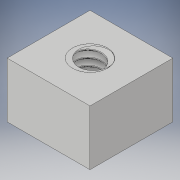
# Autodesk Inventor part: Nut0.25-20
Saved by Autodesk Inventor 2019 (Build 230136000, 136)
## iProperties
Created: 2019-08-02
Part Number: Nut0.25-20
Material: Generic
Document SubType Name: Modeling
Designer: aorfi
Density: 1 g/cm^3
Appearance: Default
Author: aorfi
Autodesk Inventor part; units mm, degrees
ref_plane "YZ Plane" through (0, 0, 0) normal (1, 0, 0) x (0, 1, 0)
ref_plane "XZ Plane" through (0, 0, 0) normal (0, 1, 0) x (-1, 0, 0)
ref_plane "XY Plane" through (0, 0, 0) normal (0, 0, 1) x (1, 0, 0)
sketch "Sketch1" plane through (0, 0, 0) normal (0, 1, 0) x (-1, 0, 0)
  line L0 (-7.5, 7.5) -> (7.5, 7.5)
  line L1 (7.5, 7.5) -> (7.5, -7.5)
  line L2 (7.5, -7.5) -> (-7.5, -7.5)
  line L3 (-7.5, -7.5) -> (-7.5, 7.5)
  line L4 (-7.5, 7.5) -> (7.5, -7.5) construction
  line L5 (7.5, 7.5) -> (-7.5, -7.5) construction
  point P0 (0, 0)
  dimension "d0" = 15
  dimension "d1" = 15
  constraints: 12 end point, 2 midpoint, 2 parallel, 1 horizontal, 1 perpendicular
  measures "d0" distance of L0.end L1.end
  measures "d1" distance of L1.end L2.end
extrude "Extrusion1" add sketch "Sketch1" along normal mid plane 10
sketch "Sketch2" plane through (0, 5, 0) normal (0, 1, 0) x (1, 0, 0)
  circle A0 centre (0, 0) radius 3.175
  dimension "d4" = 6.35
  constraints: 1 centre point, 1 coincident
  measures "d4" diameter of A0
extrude "Extrusion2" cut sketch "Sketch2" against normal blind 10
thread "Thread1" size "1/4-20 UNC" class "2B" standard "ANSI Unified Screw Threads" full length
sketch "Sketch4" plane through (0, -5, 0) normal (-1, 0, 0) x (0, 0, 1)
  line L0 (3.175, 0) -> (3.175, 10)
  line L1 (3.175, 10) -> (2.2333, 10)
  line L2 (2.2333, 10) -> (2.2333, 0)
  line L3 (2.2333, 0) -> (3.175, 0)
  line L4 (0, -3.6619) -> (0, 12.277) projected
  constraints: 8 end point
revolve "Revolution1" add sketch "Sketch4" angle 360 about axis through (0, -5, 0) along (0, 1, 0) separate body
sketch "Sketch3" plane through (0, -5, 3.175) normal (1, 0, 0) x (0, 1, 0)
  line L0 (-0.7409, -0.0644) -> (-0.6351, -0.0644) construction
  line L1 (0.1057, -0.8776) -> (-0.0001, -1.0809) construction
  line L2 (-1.2701, -1.0809) -> (-1.3759, -0.8776) construction
  line L3 (-0.5293, -0.0644) -> (-0.6351, 0.1389) construction
  line L4 (-0.6351, 0.1389) -> (-0.7409, -0.0644) construction
  line L5 (-1.2701, -1.0809) -> (-1.1643, -0.8776) construction
  line L6 (-0.5293, -0.0644) -> (-0.1059, -0.8776)
  line L7 (-1.3759, -0.8776) -> (-1.1643, -0.8776) construction
  arc A0 (-1.3759, -0.8776) -> (-1.2701, -0.9418) centre (-1.2701, -0.8225) ccw construction
  line L8 (0.1057, -0.8776) -> (-0.1059, -0.8776) construction
  line L9 (-1.2701, -1.0809) -> (-1.2701, -0.8776) construction
  line L10 (-0.0001, -1.0809) -> (-0.0001, -0.8776) construction
  line L11 (-0.6351, 0.1389) -> (-0.6351, -0.0002) construction
  line L12 (-1.2701, -0.9418) -> (-0.0001, -0.9418)
  arc A1 (-1.2701, -0.9418) -> (-1.1643, -0.8776) centre (-1.2701, -0.8225) ccw
  line L13 (-0.1059, -0.8776) -> (-0.0001, -1.0809) construction
  line L14 (-1.1643, -0.8776) -> (-0.7409, -0.0644)
  line L15 (-0.0001, -0.0002) -> (-0.0001, 0.0177)
  line L16 (-0.0001, 0.0177) -> (-0.0001, -0.0002)
  line L17 (-0.0001, -0.0002) -> (0.0334, -0.0002)
  arc A2 (-0.1059, -0.8776) -> (-0.0001, -0.9418) centre (-0.0001, -0.8225) ccw
  arc A3 (-0.0001, -0.9418) -> (0.1057, -0.8776) centre (-0.0001, -0.8225) ccw construction
  arc A4 (-0.6351, -0.0002) -> (-0.7409, -0.0644) centre (-0.6351, -0.1195) ccw
  arc A5 (-0.5293, -0.0644) -> (-0.6351, -0.0002) centre (-0.6351, -0.1195) ccw
  line L18 (-0.6351, -0.0002) -> (-0.6351, -0.0644) construction
  line L19 (-0.6351, -0.0644) -> (-0.5293, -0.0644) construction
  dimension "d9" = 55
  dimension "d10" = 0.2033
  dimension "d11" = 0.2033
  dimension "Sketch3_ThreadOffset" = 0
  dimension "Sketch3_MajorRadius" = 0.9417
  dimension "d14" = 1.27
  dimension "Sketch3_MinorRadius" = 0
  constraints: 40 end point, 12 point on circle, 10 parallel, 8 tangent, 6 centre point, 6 collinear, 2 midpoint, 2 point on line, 1 horizontal, 1 perpendicular, 3 other
  measures "d9" angle of L6 L14
  measures "d10" distance of L3.end L0.end
  measures "d11" distance of L1.end L10.end
  measures "Sketch3_ThreadOffset" distance between parallel lines of L15 L10
  measures "Sketch3_MajorRadius" distance from line of L12 L15.start
  measures "d14" distance from line of L1.end L9
  measures "Sketch3_MinorRadius" distance edge to line of A5 L17
coil "Coil1" sketch "Sketch3" operation cut axis through (0, -5, 0) along (0, 1, 0) pitch 1.2713 turns 9.864152 hand right bodies 2
equation "\"d0\" = d1"
equation "\"d9\" = d16"
equation "\"d10\" = 0.160083 * Sketch3_Pitch"
equation "\"d11\" = 0.160083 * Sketch3_Pitch"
equation "\"d14\" = Sketch3_Pitch"
equation "\"d16\" = 55deg"
equation "\"Sketch3_Pitch\" = 1.27"
body "Solid1"
body "Solid2"
